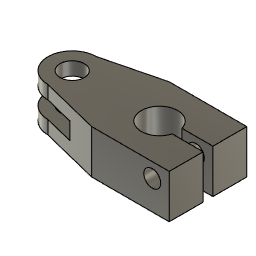
Exercise_5 v3 (Autodesk Fusion 360 design; units mm, degrees)
Autodesk Fusion 360 part; units mm, degrees
sketch "Sketch1" plane through (0, 0, 0) normal (0, 0, 1) x (1, 0, 0)
  line L0 (-16, 32) -> (16, 32)
  line L1 (16, 32) -> (16, 0)
  line L2 (16, 0) -> (-16, 0)
  line L3 (-16, 0) -> (-16, 32)
  line L4 (-16, 32) -> (16, 32)
  line L5 (16, 32) -> (16, 0)
  line L6 (-16, 0) -> (-16, 32)
  line L7 (-16, 0) -> (16, 0)
  line L8 (0, 32) -> (0, 0)
  line L9 (-10, 0) -> (10, 0)
  line L10 (10, 0) -> (10, -34)
  line L11 (10, -34) -> (-10, -34)
  line L12 (-10, -34) -> (-10, 0)
  circle A0 centre (0, -24) radius 5
  line L13 (16, 0) -> (10, -24)
  line L14 (-16, 0) -> (-10, -24)
  circle A1 centre (0, 12) radius 7.5
  line L15 (-2, 32) -> (2, 32)
  line L16 (2, 32) -> (2, 12)
  line L17 (2, 12) -> (-2, 12)
  line L18 (-2, 12) -> (-2, 32)
  dimension "d1" = 32
  dimension "d2" = 32
  dimension "d5" = 32
  dimension "d6" = 32
  dimension "d7" = 16
  dimension "d9" = 20
  dimension "d10" = 34
  dimension "d11" = 6
  dimension "d12" = 10
  dimension "d13" = 24
  dimension "d14" = 15
  dimension "d15" = 20
  dimension "d16" = 4
  dimension "d17" = 20
  dimension "d18" = 2
  constraint horizontal L0
  constraint vertical L1
  constraint horizontal L2
  constraint vertical L3
  constraint horizontal L4
  constraint vertical L5
  constraint vertical L6
  constraint coincident L1 L2.start
  constraint coincident L6 L2.end
  constraint perpendicular L5 L7
  constraint midpoint L4 L8.start
  constraint midpoint L2 L8.end
  constraint horizontal L9
  constraint vertical L10
  constraint horizontal L11
  constraint vertical L12
  constraint coincident L2 L9.start
  constraint coincident L10 L13.end
  constraint symmetric L1.end L8 L2.end
  constraint symmetric L8 L13.end L14.end
  constraint coincident L8 A1.centre
  constraint horizontal L15
  constraint vertical L16
  constraint horizontal L17
  constraint vertical L18
  constraint coincident L4 L15.start
  measures "d1" distance of L0.start L0.end
  measures "d2" distance of L0.start L2.end
  measures "d5" distance of L2.end L1.end
  measures "d6" distance of L0 L1.end
  measures "d7" distance of L8.end L1
  measures "d9" distance of L9.start L9.end
  measures "d10" distance of L9.end L10.end
  measures "d11" distance of L2.end L12
  measures "d12" diameter of A0
  measures "d13" distance of L9 A0.centre
  measures "d14" diameter of A1
  measures "d15" distance of L0 A1.centre
  measures "d16" distance of L15.start L15.end
  measures "d17" distance of L15.end L16.end
  measures "d18" distance of L8.end L16
extrude "Extrude1" add sketch "Sketch1" along normal blind 6 and the other way blind 12 contours L0 L2 L3 L4 L6 L7 L8 L9 A1 L18 | L2 L7 L12 L14 | L2 L7 L9 L10 L11 L12 | L0 L1 L2 L4 L5 L7 L8 L9 A1 L16 | L2 L7 L10 L13
sketch "Sketch2" plane through (16, 0, 0) normal (1, 0, 0) x (0, 1, 0)
  line L0 (32, -12) -> (32, 6)
  line L1 (32, 6) -> (0, 6)
  line L2 (0, 6) -> (0, -12)
  line L3 (0, -12) -> (32, -12)
  circle A0 centre (25, 0) radius 3.5
  dimension "d25" = 7
  dimension "d26" = 7
  dimension "d27" = 6
  measures "d25" diameter of A0
  measures "d26" distance of L0 A0.centre
  measures "d27" distance of L1 A0.centre
extrude "Extrude2" cut sketch "Sketch2" against normal up to surface (32 mm away) contours A0
ref_plane "WorkPlane1" through (0, -12, -3) normal (0, -1, 0) x (1, 0, 0)
sketch "Sketch3" plane through (0, -12, 0) normal (0, -1, 0) x (-1, 0, 0)
  line L0 (16, -0.5) -> (-16, -0.5)
  line L1 (-16, -0.5) -> (-16, 6.5)
  line L2 (-16, 6.5) -> (16, 6.5)
  line L3 (16, 6.5) -> (16, -0.5)
  line L4 (-10, -6) -> (-16, -6)
  dimension "d31" = 7
  dimension "d32" = 5.5
  constraint horizontal L0
  constraint vertical L1
  constraint horizontal L2
  constraint vertical L3
  measures "d31" distance of L0.end L1.end
  measures "d32" distance of L0.end L4
extrude "Extrude3" cut sketch "Sketch3" along normal up to surface (22 mm away)
fillet "Fillet2" radius 10 4 edges at (10, -34, 3.25) (-10, -34, 3.25) (-10, -34, -9.25) (10, -34, -9.25)
sketch "Sketch4" plane through (0, 0, 0) normal (1, 0, 0) x (0, 1, 0)
  line L0 (0, 32) -> (0, -24)
  constraint vertical L0
move_body "Move1" bodies 1 to x (0, -1, 0) y (1, 0, 0) z (0, 0, 1) at (0, 0, 0)
equation "d7 = ( 32 / 2 ) * 1 mm"
equation "d21 = 18 mm - 6 mm"
equation "d30 = -10 mm - 12 mm"
equation "d32 = ( ( 18 - 7 ) / 2 ) * 1 mm"
